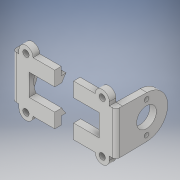
# Autodesk Inventor part: Motor mount
Saved by Autodesk Inventor 2019 (Build 230136000, 136)
## iProperties
Created: 2019-04-05
Part Number: Motor mount
Material: Generic
Document SubType Name: Modeling
Designer: jonas
Density: 1 g/cm^3
Appearance: Default
Author: jonas
Autodesk Inventor part; units mm, degrees
ref_plane "XZ Plane" through (0, 0, 0) normal (0, 1, 0) x (-1, 0, 0)
ref_plane "XY Plane" through (0, 0, 0) normal (0, 0, 1) x (1, 0, 0)
sketch "Sketch1" plane through (0, 0, 0) normal (0, 0, 1) x (1, 0, 0)
  line L0 (19, 13.5) -> (19, -13.5)
  line L1 (-19, -13.5) -> (-19, 13.5)
  line L2 (0, -24.15) -> (0, 24.15) projected
  line L3 (-26.6, 0) -> (26.6, 0) projected
  arc A0 (-11.5, 13.5) -> (-19, 13.5) centre (-15.25, 13.5) ccw
  arc A1 (-19, -13.5) -> (-11.5, -13.5) centre (-15.25, -13.5) ccw
  arc A2 (11.5, -13.5) -> (19, -13.5) centre (15.25, -13.5) ccw
  arc A3 (19, 13.5) -> (11.5, 13.5) centre (15.25, 13.5) ccw
  line L4 (-11.5, 13.5) -> (11.5, 13.5)
  line L5 (11.5, -13.5) -> (-11.5, -13.5)
  circle A4 centre (-15.25, 13.5) radius 1.65
  circle A5 centre (15.25, 13.5) radius 1.65
  circle A6 centre (15.25, -13.5) radius 1.65
  circle A7 centre (-15.25, -13.5) radius 1.65
  point P0 (0, 0)
  point P1 (-19, 0)
  point P2 (19, 0)
  dimension "d1" = 38
  dimension "d3" = 7.5
  dimension "d4" = 27
  dimension "d5" = 27
  dimension "d6" = 27
  dimension "d7" = 3.3
  constraints: 8 centre point, 8 end point, 8 point on circle, 6 equal radius, 4 coincident, 4 point on line, 4 tangent, 2 midpoint, 2 parallel, 1 horizontal, 1 perpendicular, 2 other
  measures "d1" distance between parallel lines of L0 L1
  measures "d3" diameter of A0
  measures "d4" distance between parallel lines of L5 L4
  measures "d5" distance of L1.start L1.end
  measures "d6" distance of L0.start L0.end
  measures "d7" diameter of A4
ref_plane "Work Plane1" through (19, 0, 0) normal (1, 0, 0) x (0, 1, 0)
ref_plane "Work Plane2" through (-19, 0, 0) normal (1, 0, 0) x (0, 1, 0)
sketch "Sketch3" plane through (19, 0, 0) normal (1, 0, 0) x (0, 1, 0)
  line L0 (-6.3559, 0) -> (6.3559, 0)
  line L1 (-16.1, 0) -> (16.1, 0) projected
  circle A0 centre (0, -12.73) radius 5.25
  line L2 (11.5, 0) -> (-11.5, 0)
  line L3 (11.5, 0) -> (11.2357, -12.9591)
  line L4 (-11.5, 0) -> (-11.2357, -12.9591)
  arc A1 (-11.2357, -12.9591) -> (11.2357, -12.9591) centre (0, -12.73) ccw
  line L5 (0, -29.4617) -> (0, 8.9936) projected
  circle A2 centre (8.25, -12.73) radius 1.2
  arc A3 (-11.2357, -12.9591) -> (11.2357, -12.9591) centre (0, -12.73) ccw
  circle A4 centre (-8.25, -12.73) radius 1.2
  line L6 (11.5, 0) -> (-11.5, 0)
  line L7 (-11.5, 0) -> (-11.5, 3.5)
  line L8 (-11.5, 3.5) -> (11.5, 3.5)
  line L9 (11.5, 3.5) -> (11.5, 0)
  point P0 (0, 0)
  dimension "d12" = 10.5
  dimension "d13" = 23
  dimension "d14" = 12.73
  dimension "d15" = 2.4
  dimension "d16" = 16.5
  dimension "d21" = 3.5
  constraints: 16 end point, 5 centre point, 4 point on circle, 3 symmetric about line, 2 collinear, 2 horizontal, 2 parallel, 2 tangent, 1 concentric, 1 horizontal alignment, 1 perpendicular, 3 other
  measures "d12" diameter of A0
  measures "d13" distance of L2.end L2.start
  measures "d14" distance of point (0, 0) A0.centre
  measures "d15" diameter of A2
  measures "d16" distance of A4.centre A2.centre
  measures "d21" distance between parallel lines of L2 L8
sketch "Sketch4" plane through (-19, 0, 0) normal (1, 0, 0) x (0, 1, 0)
  line L0 (0, -15.7142) -> (0, 5.0351) projected
  arc A0 (9.2431, -2.5702) -> (5.1479, 0) centre (0, -12.75) ccw
  line L1 (-9.2431, 0) -> (-9.2431, -2.5702)
  line L2 (9.2431, 0) -> (9.2431, -2.5702)
  line L3 (-13.4069, 0) -> (13.1509, 0) projected
  line L4 (-9.2431, 0) -> (-5.1479, 0)
  line L5 (-9.2431, 0) -> (-5.1479, 0)
  line L6 (-5.1479, 0) -> (9.2431, 0)
  arc A1 (5.1479, 0) -> (-9.2431, -2.5702) centre (0, -12.75) ccw
  line L7 (5.1479, 0) -> (9.2431, 0)
  line L8 (-5.1479, 0) -> (5.1479, 0)
  point P0 (-0.0291, 1)
  point P1 (13.1509, 0)
  dimension "d26" = 27.5
  dimension "d27" = 1
  constraints: 14 end point, 8 point on circle, 5 horizontal, 2 centre point, 2 horizontal alignment, 1 vertical, 4 other
  measures "d26" diameter of A0
extrude "Extrusion1" add sketch "Sketch1" along normal blind 3.5
extrude "Extrusion2" add sketch "Sketch3" along normal blind 3.5 contours L1 L7 L8 L5 L0 | L0 L5 A0 A1 L4 L1 | L5 L8 L9 L1 L0 | L0 L1 L3 A1 L5 A0
sketch "Sketch5" plane through (-19, 0, 0) normal (1, 0, 0) x (0, 1, 0)
  line L0 (0, -15.7142) -> (0, 5.0351)
  arc A0 (9.2431, -2.5702) -> (5.1479, 0) centre (0, -12.75) ccw
  line L1 (-9.2431, 0) -> (-9.2431, -2.5702)
  line L2 (9.2431, 0) -> (9.2431, -2.5702)
  line L3 (-13.4069, 0) -> (13.1509, 0)
  line L4 (-9.2431, 0) -> (-5.1479, 0)
  line L5 (-9.2431, 0) -> (-5.1479, 0)
  line L6 (-5.1479, 0) -> (9.2431, 0)
  arc A1 (5.1479, 0) -> (-9.2431, -2.5702) centre (0, -12.75) ccw
  line L7 (5.1479, 0) -> (9.2431, 0)
  line L8 (-5.1479, 0) -> (5.1479, 0)
  point P0 (0, 0)
  point P1 (-0.0291, 1)
  point P2 (13.1509, 0)
  dimension "d28" = 27.5
  dimension "d29" = 1
  constraints: 14 end point, 8 point on circle, 5 horizontal, 2 centre point, 2 horizontal alignment, 1 vertical, 8 other
  measures "d28" diameter of A0
extrude "Extrusion3" add sketch "Sketch5" along normal blind 38 contours A1 L1 L3 | L3 L2 A0
extrude "Extrusion4" cut sketch "Sketch4" along normal blind 38 contours L3 A1 L0 | L0 A1 L3
fillet "Fillet1" radius 2 1 edges at (22.5, 0, 3.5)
sketch "Sketch6" plane through (0, 0, 3.5) normal (0, 0, 1) x (1, 0, 0)
  line L0 (-13.6102, -5.8026) -> (13.6102, -5.8026)
  line L1 (13.6102, -5.8026) -> (13.6102, 5.8026)
  line L2 (13.6102, 5.8026) -> (-13.6102, 5.8026)
  line L3 (-13.6102, 5.8026) -> (-13.6102, -5.8026)
  line L4 (-27.3, 0) -> (30.8, 0) projected
  line L5 (0, -24.15) -> (0, 24.15) projected
  point P0 (0, 0)
  constraints: 8 end point, 2 parallel, 1 horizontal, 1 perpendicular, 2 other
extrude "Extrusion5" cut sketch "Sketch6" against normal blind 38
sketch "Sketch7" plane through (-19, 0, 0) normal (1, 0, 0) x (0, 1, 0)
  line L0 (11.5, 3.5) -> (-11.5, 3.5)
  line L1 (0, -16.9401) -> (0, 12.391) projected
  circle A0 centre (0, -5.2) radius 1.1
  line L2 (-11.5, 0) -> (11.5, 0)
  line L3 (11.5, -3.9814) -> (8.6809, -3.9814)
  line L4 (-11.5, 3.5) -> (-11.5, -3.9814)
  line L5 (11.5, 3.5) -> (11.5, -3.9814)
  arc A1 (-8.6809, -3.9814) -> (8.6809, -3.9814) centre (0, 8.2008) ccw
  line L6 (-8.6809, -3.9814) -> (-11.5, -3.9814)
  arc A2 (9.2431, -2.5702) -> (-9.2431, -2.5702) centre (0, -12.75) ccw projected
  point P0 (0, 0)
  point P1 (0, 1)
  dimension "d39" = 2.2
  dimension "d40" = 6.2
  dimension "d41" = 23
  dimension "d48" = 3.5
  constraints: 12 end point, 3 point on circle, 3 point on line, 2 centre point, 2 horizontal, 2 parallel, 2 perpendicular
  measures "d39" diameter of A0
  measures "d40" distance of point (0, 1) A0.centre
  measures "d41" distance of L3.start L4.end
  measures "d48" distance between parallel lines of L0 L2
extrude "Extrusion6" add sketch "Sketch7" against normal blind 3.5 contours L5 L2 A2 L1 L0 | L1 A2 L2 L4 L0 | L5 L3 A1 L1 A0 L2 | A2 L2 L1 | L1 L2 A2 | L2 L1 A0 A1 L6 L4
split body "Split2" result two bodies by plane through (0, 0, 0) normal (1, 0, 0) first body at (22, -0.2109, -1.5061)
move or copy body "Move Body1" bodies to move or copy 2 copy no translate (10, 0, 0)
fillet "Fillet2" radius 2 1 edges at (-22.5, 0, 3.5)
equation "\"d5\" = d4"
equation "\"d6\" = d4"
body "Solid2"
body "Solid3"
